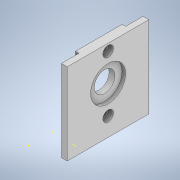
# Autodesk Inventor part: 220307 Rod Support Part B Corrected
Saved by Autodesk Inventor 2022 (Build 260153000, 153)
## iProperties
Created: 2022-01-10
Part Number: 220307 Rod Support Part B Corrected
Material: Generic
Document SubType Name: Modeling
Designer: josephinew
Density: 1 g/cm^3
Appearance: Default
Author: josephinew
Autodesk Inventor part; units mm, degrees
ref_plane "YZ Plane" through (0, 0, 0) normal (1, 0, 0) x (0, 1, 0)
ref_plane "XZ Plane" through (0, 0, 0) normal (0, 1, 0) x (-1, 0, 0)
ref_plane "XY Plane" through (0, 0, 0) normal (0, 0, 1) x (1, 0, 0)
sketch "Sketch3" plane through (0, 0, 0) normal (1, 0, 0) x (0, 1, 0)
  line L0 (0, 0) -> (76.2, 0)
  line L1 (76.2, 0) -> (76.2, -76.2)
  line L2 (76.2, -76.2) -> (0, -76.2)
  line L3 (0, -76.2) -> (0, 0)
  line L4 (76.2, 0) -> (50.8, 0)
  line L5 (50.8, 50.8) -> (76.2, 50.8)
  line L6 (76.2, 50.8) -> (76.2, 0)
  line L7 (76.2, -76.2) -> (50.8, -76.2)
  line L8 (50.8, -127) -> (76.2, -127)
  line L9 (76.2, -127) -> (76.2, -76.2)
  line L10 (50.8, 50.8) -> (-50.8, 50.8)
  line L11 (-50.8, 50.8) -> (-50.8, 0)
  line L12 (0, 0) -> (50.8, 0)
  line L13 (50.8, -76.2) -> (0, -76.2)
  line L14 (-50.8, -76.2) -> (-50.8, -127)
  line L15 (-50.8, -127) -> (50.8, -127)
  line L16 (0, 0) -> (0, -76.2)
  line L17 (-50.8, -76.2) -> (-50.8, 0)
  dimension "d1" = 76.2
  dimension "d26" = 50.8
  constraints: 36 end point, 7 parallel, 5 horizontal, 3 perpendicular, 1 point on line
  measures "d1" distance of L0.end L1.end
  measures "d26" distance of L14.end L14.start
extrude "Extrusion1" add sketch "Sketch3" along normal blind 25.4
sketch "Sketch5" plane through (0, 0, 0) normal (-1, 0, 0) x (0, 0, 1)
  line L0 (-76.2, 76.2) -> (0, 76.2) projected
  line L1 (-76.2, 76.2) -> (-38.1, 76.2)
  line L2 (-38.1, 76.2) -> (-38.1, 63.5)
  line L3 (-38.1, 63.5) -> (-38.1, 38.1)
  circle A0 centre (-38.1, 38.1) radius 11.2522
  point P0 (0, 0)
  dimension "d10" = 38.1
  dimension "d11" = 12.7
  dimension "d12" = 25.4
  dimension "d13" = 22.5044
  constraints: 6 end point, 1 centre point, 1 coincident, 1 midpoint, 1 perpendicular, 1 point on line
  measures "d10" distance of L0.start L1.end
  measures "d11" distance of L1.end L2.end
  measures "d12" distance of L2.end L3.end
  measures "d13" diameter of A0
extrude "Extrusion3" cut sketch "Sketch5" against normal blind 76.2
sketch "Sketch6" plane through (25.4, 0, 0) normal (1, 0, 0) x (0, 0, -1)
  circle A0 centre (38.1, 38.1) radius 11.2522 projected
  circle A1 centre (38.1, 38.1) radius 19.05
  point P0 (0, 0)
  dimension "d20" = 38.1
  constraints: 1 centre point, 1 coincident
  measures "d20" diameter of A1
extrude "Extrusion4" cut sketch "Sketch6" against normal blind 6.35
sketch "Sketch8" plane through (0, 76.2, 50.8) normal (0, 1, 0) x (1, 0, 0)
  line L0 (0, 0) -> (25.4, 0) projected
  line L1 (12.7, 0) -> (9.525, 0)
  line L2 (9.525, 0) -> (15.875, 0)
  line L3 (15.875, 0) -> (15.875, 50.8)
  line L4 (15.875, 50.8) -> (9.525, 50.8)
  line L5 (9.525, 50.8) -> (9.525, 0)
  line L6 (0, 177.8) -> (0, 0) projected
  line L7 (12.7, 177.8) -> (9.525, 177.8)
  line L8 (9.525, 177.8) -> (15.875, 177.8)
  line L9 (15.875, 177.8) -> (15.875, 127)
  line L10 (15.875, 127) -> (9.525, 127)
  line L11 (9.525, 127) -> (9.525, 177.8)
  line L12 (0, 0) -> (0, 177.8)
  point P0 (0, 50.8)
  point P1 (25.4, 177.8)
  point P2 (15.875, 0)
  dimension "d28" = 6.35
  dimension "d29" = 50.8
  constraints: 22 end point, 2 parallel, 1 horizontal, 1 midpoint, 1 perpendicular, 1 point on line
  measures "d28" distance of L4.end L3.end
  measures "d29" distance of L3.end L2.end
extrude "Extrusion5" cut sketch "Sketch8" against normal blind 76.2
sketch "Sketch9" plane through (0, -50.8, 50.8) normal (0, 0, 1) x (1, 0, 0)
  line L0 (9.525, 50.8) -> (15.875, 50.8)
  line L1 (15.875, 50.8) -> (15.875, 0)
  line L2 (15.875, 0) -> (9.525, 0)
  line L3 (9.525, 0) -> (9.525, 50.8)
  point P0 (0, 50.8)
  dimension "d32" = 6.35
  dimension "d33" = 50.8
  constraints: 8 end point, 2 parallel, 1 horizontal, 1 perpendicular
  measures "d32" distance of L1.end L2.end
  measures "d33" distance of L0.end L1.end
extrude "Extrusion6" cut sketch "Sketch9" against normal blind 203.2
sketch "Sketch10" plane through (0, 0, 0) normal (-1, 0, 0) x (0, 0, 1)
  circle A0 centre (-38.1, 38.1) radius 11.2522 projected
  circle A1 centre (-38.1, 38.1) radius 19.05
  point P0 (0, 0)
  dimension "d36" = 38.1
  constraints: 1 centre point, 1 coincident
  measures "d36" diameter of A1
extrude "Extrusion7" cut sketch "Sketch10" against normal blind 5.08 contours A0 | A1
sketch "Sketch11" plane through (0, 76.2, 50.8) normal (0, 1, 0) x (1, 0, 0)
  line L0 (9.525, 50.8) -> (15.875, 50.8) projected
  line L1 (16.51, 50.8) -> (16.51, 0)
  line L2 (16.51, 0) -> (8.89, 0)
  line L3 (9.525, 177.8) -> (9.525, 0) projected
  line L4 (8.89, 0) -> (8.89, 51.308)
  line L5 (8.89, 0) -> (60.198, 0) construction
  line L6 (8.89, 51.308) -> (16.51, 51.308)
  line L7 (16.51, 51.308) -> (16.51, 50.8)
  line L8 (0, 69.85) -> (0, 107.95) projected
  line L9 (0, 88.9) -> (23.8125, 88.9)
  line L10 (9.525, 127) -> (15.875, 127)
  line L11 (16.51, 127) -> (16.51, 177.8)
  line L12 (16.51, 177.8) -> (8.89, 177.8)
  line L13 (8.89, 177.8) -> (8.89, 126.492)
  line L14 (8.89, 126.492) -> (16.51, 126.492)
  line L15 (16.51, 126.492) -> (16.51, 127)
  point P0 (0, 50.8)
  point P1 (0, 127)
  dimension "d40" = 7.62
  constraints: 26 end point, 8 symmetric about line, 3 perpendicular, 2 horizontal, 1 midpoint, 1 vertical
  measures "d40" distance of L1.end L2.end
extrude "Extrusion8" cut sketch "Sketch11" against normal blind 152.4
sketch "Sketch12" plane through (25.4, -50.8, 50.8) normal (0, 0, 1) x (1, 0, 0)
  line L0 (-8.89, 127) -> (-8.89, 0) projected
  line L1 (-16.51, 127) -> (-16.51, 0) projected
  line L2 (-8.89, 50.8) -> (-16.51, 50.8)
  line L3 (-16.51, 50.8) -> (-16.51, 0)
  line L4 (-16.51, 0) -> (-8.89, 0)
  line L5 (-8.89, 0) -> (-8.89, 50.8)
  point P0 (-25.4, 50.8)
  constraints: 8 end point, 2 parallel, 1 horizontal, 1 perpendicular, 1 point on line
extrude "Extrusion9" cut sketch "Sketch12" against normal blind 203.2
sketch "Sketch13" plane through (25.4, 0, 0) normal (1, 0, 0) x (0, 0, -1)
  line L0 (127, 76.2) -> (-50.8, 76.2) projected
  line L1 (-50.8, -50.8) -> (127, -50.8) projected
  line L2 (-50.8, 76.2) -> (-25.4, 76.2)
  line L3 (-25.4, 76.2) -> (-25.4, -50.8)
  line L4 (-25.4, -50.8) -> (-50.8, -50.8)
  line L5 (-50.8, -50.8) -> (-50.8, 76.2)
  line L6 (127, -50.8) -> (127, 76.2) projected
  line L7 (127, 76.2) -> (75.692, 76.2) projected
  line L8 (127, -50.8) -> (101.6, -50.8)
  line L9 (101.6, -50.8) -> (101.6, 76.2)
  line L10 (101.6, 76.2) -> (127, 76.2)
  line L11 (127, 76.2) -> (127, -50.8)
  point P0 (0, 0)
  dimension "d49" = 25.4
  dimension "d50" = 25.4
  constraints: 16 end point, 4 parallel, 2 horizontal, 2 perpendicular, 2 point on line
  measures "d49" distance of L3.end L4.end
  measures "d50" distance of L9.end L10.end
extrude "Extrusion10" cut sketch "Sketch13" against normal blind 25.4 contours L6 L1 L9 L0 | L3 L1 L5 L0
sketch "Sketch14" plane through (25.4, 0, 0) normal (1, 0, 0) x (0, 0, -1)
  line L0 (-25.4, -50.8) -> (101.6, -50.8) projected
  line L1 (101.6, -50.8) -> (101.6, 76.2) projected
  line L2 (-25.4, -50.8) -> (101.6, -50.8)
  line L3 (101.6, -50.8) -> (101.6, -12.7)
  line L4 (101.6, -12.7) -> (-25.4, -12.7)
  line L5 (-25.4, -12.7) -> (-25.4, -50.8)
  point P0 (0, 0)
  dimension "d53" = 38.1
  constraints: 8 end point, 2 parallel, 1 horizontal, 1 perpendicular, 1 point on line
  measures "d53" distance of L3.end L2.end
extrude "Extrusion11" cut sketch "Sketch14" against normal blind 25.4
sketch "Sketch15" plane through (25.4, 0, 0) normal (1, 0, 0) x (0, 0, -1)
  point P0 (0, 0)
sketch "Sketch16" plane through (0, 76.2, 25.4) normal (0, 0, 1) x (1, 0, 0)
  point P0 (0, -76.2)
sketch "Sketch17" plane through (8.89, 76.2, -75.692) normal (0, 1, 0) x (1, 0, 0)
  line L0 (-8.89, -101.092) -> (0, -101.092) projected
  line L1 (7.62, 25.908) -> (7.62, -101.092) projected
  line L2 (0, -101.092) -> (7.62, -101.092)
  line L3 (7.62, -101.092) -> (7.62, -62.992)
  line L4 (7.62, -62.992) -> (0, -62.992)
  line L5 (0, -62.992) -> (0, -101.092)
  line L6 (7.62, 25.908) -> (7.62, 0) projected
  line L7 (0, -101.092) -> (0, 25.908) projected
  line L8 (7.62, 25.908) -> (0, 25.908)
  line L9 (0, 25.908) -> (0, -12.192)
  line L10 (0, -12.192) -> (7.62, -12.192)
  line L11 (7.62, -12.192) -> (7.62, 25.908)
  point P0 (-8.89, -75.692)
  point P1 (7.62, -12.192)
  dimension "d56" = 38.1
  dimension "d57" = 38.1
  constraints: 16 end point, 4 parallel, 2 horizontal, 2 perpendicular, 2 point on line
  measures "d56" distance of L3.end L2.end
  measures "d57" distance of L9.end L8.end
extrude "Extrusion12" cut sketch "Sketch17" against normal blind 76.2 contours L1 L10 L7 L8 | L1 L2 L5 L4
sketch "Sketch18" plane through (8.89, 0, -12.7) normal (0, -1, 0) x (1, 0, 0)
  point P0 (-8.89, 12.7)
sketch "Sketch19" plane through (25.4, 0, 0) normal (1, 0, 0) x (0, 0, -1)
  line L0 (12.7, 76.2) -> (-25.4, 76.2) projected
  line L1 (-25.4, -12.7) -> (-6.35, -12.7)
  line L2 (-6.35, -12.7) -> (-6.35, 76.2)
  line L3 (-6.35, 76.2) -> (-25.4, 76.2)
  line L4 (-25.4, 76.2) -> (-25.4, -12.7)
  line L5 (101.6, -12.7) -> (-25.4, -12.7) projected
  line L6 (101.6, 76.2) -> (-25.4, 76.2) projected
  line L7 (101.6, -12.7) -> (82.55, -12.7)
  line L8 (82.55, -12.7) -> (82.55, 76.2)
  line L9 (82.55, 76.2) -> (101.6, 76.2)
  line L10 (101.6, 76.2) -> (101.6, -12.7)
  point P0 (0, 0)
  dimension "d60" = 19.05
  constraints: 16 end point, 4 parallel, 2 horizontal, 2 perpendicular, 1 midpoint, 1 point on line
  measures "d60" distance of L8.end L9.end
extrude "Extrusion13" cut sketch "Sketch19" against normal blind 76.2 contours L2 L1 L4 L0 | L6 L10 L5 L8
sketch "Sketch20" plane through (0, 76.2, 6.35) normal (0, 0, 1) x (1, 0, 0)
  line L0 (8.89, -88.9) -> (0, -88.9) projected
  line L1 (8.89, 0) -> (8.89, -76.2) projected
  line L2 (0, -88.9) -> (8.89, -88.9)
  line L3 (8.89, -88.9) -> (8.89, 0)
  line L4 (8.89, 0) -> (0, 0)
  line L5 (0, 0) -> (0, -88.9)
  point P0 (0, -76.2)
  constraints: 8 end point, 2 parallel, 1 horizontal, 1 perpendicular
extrude "Extrusion14" cut sketch "Sketch20" against normal blind 127
sketch "Sketch21" plane through (25.4, 0, 0) normal (1, 0, 0) x (0, 0, -1)
  point P0 (0, 0)
sketch "Sketch22" plane through (16.51, 76.2, 6.35) normal (0, 1, 0) x (1, 0, 0)
  line L0 (0, 19.05) -> (-7.62, 19.05) projected
  line L1 (-7.62, 69.85) -> (0, 69.85) projected
  line L2 (0, 19.05) -> (-3.175, 19.05)
  line L3 (-3.175, 19.05) -> (-3.175, 69.85)
  line L4 (-3.175, 69.85) -> (0, 69.85)
  line L5 (0, 69.85) -> (0, 19.05)
  line L6 (-7.62, 69.85) -> (-7.62, 19.05) projected
  line L7 (-3.175, 69.85) -> (-7.62, 69.85)
  line L8 (-7.62, 69.85) -> (-7.62, 19.05)
  line L9 (-7.62, 19.05) -> (-3.175, 19.05)
  line L10 (-3.175, 19.05) -> (-3.175, 69.85)
  point P0 (-16.51, 6.35)
  point P1 (-3.175, 19.05)
  dimension "d65" = 3.175
  constraints: 16 end point, 4 parallel, 2 horizontal, 2 perpendicular, 1 point on line
  measures "d65" distance of L3.end L4.end
extrude "Extrusion15" cut sketch "Sketch22" against normal blind 127 contours L0 L6 L1 L3
sketch "Sketch23" plane through (25.4, -12.7, 6.35) normal (0, 0, 1) x (1, 0, 0)
  line L0 (0, 88.9) -> (-8.89, 88.9) projected
  line L1 (-8.89, 0) -> (-2.54, 0)
  line L2 (-2.54, 0) -> (-2.54, 88.9)
  line L3 (-2.54, 88.9) -> (-8.89, 88.9)
  line L4 (-8.89, 88.9) -> (-8.89, 0)
  line L5 (-2.54, 88.9) -> (0, 88.9)
  line L6 (0, 88.9) -> (0, 0)
  line L7 (0, 0) -> (-2.54, 0)
  line L8 (-2.54, 0) -> (-2.54, 88.9)
  point P0 (-25.4, 12.7)
  dimension "d68" = 6.35
  constraints: 16 end point, 4 parallel, 2 horizontal, 2 perpendicular, 1 point on line
  measures "d68" distance of L3.end L2.end
extrude "Extrusion16" cut sketch "Sketch23" against normal blind 127 contours L6 L7 L2 L0
sketch "Sketch24" plane through (22.86, -12.7, 6.35) normal (1, 0, 0) x (0, 0, -1)
  circle A0 centre (44.45, 50.8) radius 19.05 projected
  circle A1 centre (44.45, 81.28) radius 3.175
  circle A2 centre (44.45, 20.32) radius 3.175
  point P0 (6.35, 12.7)
  dimension "d72" = 6.35
  dimension "d74" = 6.35
  constraints: 2 centre point
  measures "d72" diameter of A1
  measures "d74" diameter of A2
extrude "Extrusion17" cut sketch "Sketch24" against normal blind 127 contours A1 | A2
sketch "Sketch25" plane through (22.86, -12.7, 6.35) normal (1, 0, 0) x (0, 0, -1)
  circle A0 centre (44.45, 81.28) radius 3.175 projected
  circle A1 centre (44.45, 81.28) radius 5.715
  circle A2 centre (44.45, 20.32) radius 3.175 projected
  circle A3 centre (44.45, 20.32) radius 5.715
  point P0 (6.35, 12.7)
  dimension "d77" = 11.43
  dimension "d78" = 11.43
  constraints: 2 centre point, 2 coincident
  measures "d77" diameter of A1
  measures "d78" diameter of A3
extrude "Extrusion18" cut sketch "Sketch25" against normal blind 5.08 contours A0 | A1 | A2 | A3
sketch "Sketch26" plane through (13.335, 76.2, -63.5) normal (-1, 0, 0) x (0, 0, 1)
  point P0 (63.5, -76.2)
sketch "Sketch27" plane through (22.86, -12.7, 6.35) normal (1, 0, 0) x (0, 0, -1)
  point P0 (6.35, 12.7)
sketch "Sketch28" plane through (13.335, 76.2, -63.5) normal (-1, 0, 0) x (0, 0, 1)
  point P0 (63.5, -76.2)
sketch "Sketch30" plane through (13.335, 76.2, -63.5) normal (-1, 0, 0) x (0, 0, 1)
  circle A0 centre (25.4, -7.62) radius 3.175 projected
  circle A1 centre (25.4, -7.62) radius 3.175
  circle A2 centre (25.4, -38.1) radius 11.2522 projected
  circle A3 centre (25.4, -38.1) radius 11.2522
  circle A4 centre (25.4, -68.58) radius 3.175 projected
  circle A5 centre (25.4, -68.58) radius 3.175
  line L0 (0, -76.2) -> (50.8, -76.2)
  line L1 (50.8, -76.2) -> (50.8, 0)
  line L2 (50.8, 0) -> (0, 0)
  line L3 (0, 0) -> (0, -76.2)
  point P0 (63.5, -76.2)
  constraints: 8 end point, 3 centre point, 3 coincident, 2 parallel, 1 horizontal, 1 perpendicular
extrude "Extrusion19" add sketch "Sketch30" along normal blind 0.635
body "Solid1"
